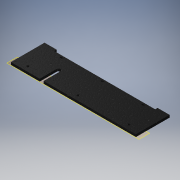
# Autodesk Inventor part: sides-02
Saved by Autodesk Inventor 2018 (Build 220112000, 112)
## iProperties
Created: 2017-10-09
Part Number: sides-02
Material: Generic
Document SubType Name: Modeling
Designer: HP
Density: 1 g/cm^3
Appearance: Fine Textured - Black
Author: HP
Autodesk Inventor part; units mm, degrees
ref_plane "YZ Plane" through (0, 0, 0) normal (1, 0, 0) x (0, 1, 0)
ref_plane "XZ Plane" through (0, 0, 0) normal (0, 1, 0) x (-1, 0, 0)
ref_plane "XY Plane" through (0, 0, 0) normal (0, 0, 1) x (1, 0, 0)
ref_plane "Work Plane1" through (0, 0, 0) normal (0, 0, 1) x (1, 0, 0)
sketch "Sketch1" plane through (0, 0, 0) normal (0, 0, 1) x (1, 0, 0)
  line L0 (250, 0) -> (0, 0) construction
  line L1 (250, 0) -> (250, 20) construction
  line L2 (0, 20) -> (250, 20) construction
  line L3 (0, 0) -> (0, 20) construction
  line L4 (245, 20) -> (153.1686, 20) construction
  line L5 (245, 20) -> (245, 80) construction
  line L6 (153.1686, 80) -> (245, 80) construction
  line L7 (153.1686, 20) -> (153.1686, 80) construction
  line L8 (-5, 0) -> (255, 0)
  line L9 (255, 0) -> (255, 70)
  line L10 (255, 70) -> (230, 70)
  line L11 (230, 70) -> (230, 65)
  line L12 (230, 65) -> (20, 65)
  line L13 (20, 65) -> (20, 70)
  line L14 (20, 70) -> (-5, 70)
  line L15 (-5, 70) -> (-5, 0)
  dimension "d0" = 10
  dimension "d1" = 5
  dimension "d2" = 5
  dimension "d3" = 5
  dimension "d4" = 25
  dimension "d5" = 25
  constraints: 18 end point, 5 perpendicular, 3 point on line, 1 collinear, 1 vertical
  measures "d0" distance between parallel lines of L10 L6
  measures "d1" distance between parallel lines of L12 L10
  measures "d2" distance between parallel lines of L15 L3
  measures "d3" distance between parallel lines of L9 L1
  measures "d4" distance between parallel lines of L13 L15
  measures "d5" distance between parallel lines of L11 L9
extrude "Extrusion1" add sketch "Sketch1" along normal blind 5
hole "Hole1" [suppressed]
hole "Hole2" [suppressed]
sketch "Sketch2" plane through (0, 0, 0) normal (0, 0, -1) x (-1, 0, 0)
  line L0 (0, 0) -> (-250, 0) construction
  line L1 (0, 0) -> (0, 20) construction
  line L2 (-250, 20) -> (0, 20) construction
  line L3 (-250, 0) -> (-250, 20) construction
  line L4 (5, 0) -> (-255, 0) construction
  line L5 (5, 70) -> (5, 0) construction
  line L6 (-20, 70) -> (5, 70) construction
  line L7 (-20, 65) -> (-20, 70) construction
  line L8 (-230, 65) -> (-20, 65) construction
  line L9 (-230, 70) -> (-230, 65) construction
  line L10 (-255, 70) -> (-230, 70) construction
  line L11 (-255, 0) -> (-255, 70) construction
  line L12 (-125, 20) -> (-125, 0) construction
  line L13 (-250, 10) -> (0, 10) construction
  point P0 (-125, 10)
  point P1 (-230, 10)
  point P2 (-20, 10)
  dimension "d30" = 20
  dimension "d31" = 20
  constraints: 5 midpoint, 4 end point, 2 point on line
  measures "d30" distance from line of point (-230, 10) L3
  measures "d31" distance from line of point (-20, 10) L1
hole "Hole3" at (125, 10, 0) at (230, 10, 0) at (20, 10, 0) direction (0, 0, 1) diameter 5 end through all
sketch "Sketch3" plane through (20, 65, 0) normal (0, 1, 0) x (1, 0, 0)
  line L0 (210, 0) -> (0, 0) construction
  line L1 (0, 0) -> (0, -5) construction
  line L2 (210, -5) -> (0, -5) construction
  line L3 (210, 0) -> (210, -5) construction
  line L4 (210, 0) -> (210, -5) construction
  line L5 (0, 0) -> (0, -5) construction
  line L6 (0, -2.5) -> (210, -2.5) construction
  line L7 (-25, -5) -> (235, -5) construction
  line L8 (105, -5) -> (105, 0) construction
  line L9 (-25, 0) -> (235, 0) construction
  point P0 (-20, 0)
  point P1 (105, -2.5)
  point P2 (20, -2.5)
  point P3 (190, -2.5)
  dimension "d39" = 20
  dimension "d40" = 20
  constraints: 5 midpoint, 4 end point, 2 point on line
  measures "d39" distance from line of point (190, -2.5) L3
  measures "d40" distance from line of point (20, -2.5) L1
hole "Hole4" at (125, 65, 2.5) at (40, 65, 2.5) at (210, 65, 2.5) direction (0, -1, 0) diameter 2.459 depth 8.8 tip angle 118 thread size "M3x0.5" class "6H" standard "ISO Metric profile"
sketch "Sketch4" plane through (0, 0, 5) normal (0, 0, 1) x (1, 0, 0)
  line L0 (41.2295, 56.2) -> (41.2295, 65) construction
  line L1 (38.7705, 56.2) -> (38.7705, 65) construction
  line L2 (126.2295, 56.2) -> (126.2295, 65) construction
  line L3 (123.7705, 56.2) -> (123.7705, 65) construction
  line L4 (208.7705, 56.2) -> (208.7705, 65) construction
  line L5 (211.2295, 56.2) -> (211.2295, 65) construction
  line L6 (37.15, 62) -> (42.85, 62)
  line L7 (42.85, 62) -> (42.85, 59)
  line L8 (42.85, 59) -> (37.15, 59)
  line L9 (37.15, 59) -> (37.15, 62)
  line L10 (38.7705, 65) -> (41.2295, 65) construction
  line L11 (230, 65) -> (20, 65) construction
  line L12 (40, 65) -> (40, 60.5) construction
  line L13 (122.15, 62) -> (127.85, 62)
  line L14 (127.85, 62) -> (127.85, 59)
  line L15 (127.85, 59) -> (122.15, 59)
  line L16 (122.15, 59) -> (122.15, 62)
  line L17 (123.7705, 65) -> (126.2295, 65) construction
  line L18 (125, 65) -> (125, 61.2984) construction
  line L19 (212.85, 62) -> (212.85, 59)
  line L20 (210, 65) -> (210, 58.9) construction
  line L21 (208.7705, 65) -> (211.2295, 65) construction
  line L22 (207.15, 62) -> (212.85, 62)
  line L23 (212.85, 59) -> (207.15, 59)
  line L24 (207.15, 59) -> (207.15, 62)
  point P0 (0, 0)
  dimension "d48" = 3
  dimension "d50" = 5.7
  dimension "d51" = 3
  dimension "d52" = 3
  dimension "d53" = 5.7
  dimension "d54" = 3
  dimension "d55" = 3
  dimension "d56" = 5.7
  dimension "d57" = 3
  constraints: 36 end point, 6 parallel, 5 perpendicular, 3 horizontal, 3 midpoint, 3 vertical, 2 collinear, 3 other
  measures "d48" distance between parallel lines of L8 L6
  measures "d50" distance between parallel lines of L7 L9
  measures "d51" distance between parallel lines of L6 L10
  measures "d52" distance between parallel lines of L15 L13
  measures "d53" distance between parallel lines of L14 L16
  measures "d54" distance between parallel lines of L13 L17
  measures "d55" distance between parallel lines of L23 L22
  measures "d56" distance between parallel lines of L19 L24
  measures "d57" distance between parallel lines of L22 L21
extrude "Extrusion2" cut sketch "Sketch4" against normal through all
sketch "Sketch5" plane through (0, 0, 5) normal (0, 0, 1) x (1, 0, 0)
  arc A0 (63, 35) -> (55, 35) centre (59, 35) ccw projected
  line L0 (63, 35) -> (63, 0) projected
  line L1 (55, 0) -> (55, 35) projected
  line L2 (55, 0) -> (63, 0)
  line L3 (-5, 0) -> (255, 0) projected
  point P0 (0, 0)
  constraints: 2 end point, 1 collinear
extrude "Extrusion3" [suppressed]
equation "\"d1\" = ABS_tolerance + plate_thickness"
equation "\"d2\" = plate_thickness + basic_plate_offset"
equation "\"d3\" = plate_thickness + basic_plate_offset"
equation "\"d5\" = d4"
equation "\"d6\" = plate_thickness"
equation "\"d40\" = d39"
equation "\"d52\" = d48"
equation "\"d53\" = d50"
equation "\"d55\" = d58"
equation "\"d56\" = d59"
equation "\"plate_thickness\" = 5"
equation "\"ABS_tolerance\" = 0"
equation "\"laser_cutter_thickness\" = 0.1"
equation "\"basic_plate_offser\" = 0.5"
equation "\"basic_plate_offset\" = 0"
equation "\"d58\" = 3"
equation "\"d59\" = 5.7"
body "Solid1"
